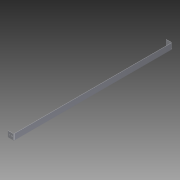
# Autodesk Inventor part: Climber Connector Bar
Saved by Autodesk Inventor 2014 SP1 (Build 180222100, 222)
## iProperties
Created: 2013-12-13
Part Number: Climber Connector Bar
Material: Aluminum 6061
Document SubType Name: Sheet Metal
Designer: Moses
Density: 2.71 g/cm^3
Appearance: Aluminum - Flat
Sheet Metal Rule: Default
Mass: 42.8559 g
Surface Area: 408.203 cm^2
Volume: 15.814 cm^3
Author: Moses
Autodesk Inventor part; units mm, degrees
ref_plane "YZ Plane" through (0, 0, 0) normal (1, 0, 0) x (0, 1, 0)
ref_plane "XZ Plane" through (0, 0, 0) normal (0, 1, 0) x (-1, 0, 0)
ref_plane "XY Plane" through (0, 0, 0) normal (0, 0, 1) x (1, 0, 0)
sketch "Sketch1" plane through (0, 0, 0) normal (0, 0, 1) x (1, 0, 0)
  line L0 (0, 0) -> (19.05, 0)
  line L1 (19.05, 0) -> (19.05, 19.05)
  line L2 (19.05, 19.05) -> (18.2563, 19.05)
  line L3 (18.2563, 19.05) -> (18.2563, 0.7938)
  line L4 (18.2563, 0.7938) -> (0, 0.7937)
  line L5 (0, 0.7937) -> (0, 0)
  dimension "d0" = 19.05
  dimension "d1" = 19.05
  dimension "d2" = 0.7937
  constraints: 12 end point, 3 horizontal, 3 vertical, 1 perpendicular
  measures "d0" distance of L0.start L0.end
  measures "d1" distance of L0.end L1.end
  measures "d2" distance of L1.end L2.end
extrude "Extrusion1" add sketch "Sketch1" along normal blind 260.35
sketch "Sketch2" plane through (0, 0, 260.35) normal (0, 0, 1) x (1, 0, 0)
  line L0 (0, 0) -> (19.05, 0) projected
  line L1 (19.05, 0) -> (19.05, 19.05) projected
  line L2 (19.05, 19.05) -> (18.2563, 19.05) projected
  line L3 (18.2563, 19.05) -> (18.2563, 0.7938) projected
  line L4 (18.2563, 0.7938) -> (18.2563, 0)
  constraints: 2 end point, 1 point on line, 1 vertical
extrude "Extrusion2" cut sketch "Sketch2" against normal blind 3.175
sketch "Sketch3" plane through (18.2563, 0, 259.5563) normal (0, 0, 1) x (1, 0, 0)
  line L0 (-18.2563, 0) -> (0, 0)
  line L1 (0, 0) -> (0, 19.05)
  line L2 (0, 19.05) -> (-18.2563, 19.05)
  line L3 (-18.2563, 19.05) -> (-18.2563, 0)
  constraints: 6 end point, 1 horizontal, 1 perpendicular, 1 vertical
edge flange "Flange1" height 19.05 angle 90 thickness 0.7937 bend radius 0.635 thickness toward (0, 0, 1) relief straight relief width 0.7937 relief depth 0.3969 edges at (9.1281, 0.7938, 260.35) wall of the first edge with corners at (0, 0, 259.5563) (18.2563, 0, 259.5563) (18.2562, 19.05, 259.5563) (0, 19.05, 259.5563)
bend "Bend1"
corner "Corner1"
sketch "Sketch4" plane through (0, 19.05, 260.35) normal (0, 0, 1) x (1, 0, 0)
  line L0 (0, -17.6213) -> (18.2563, -17.6213) projected
  line L1 (0, 0) -> (18.2563, 0) projected
  circle A0 centre (5.1594, -8.8106) radius 1.5875
  circle A1 centre (13.0969, -8.8106) radius 1.5875
  line L2 (5.1594, -8.8106) -> (13.0969, -8.8106) construction
  line L3 (9.1281, 0) -> (9.1281, -17.6213) construction
  point P0 (0, -19.05)
  point P1 (9.1281, -8.8106)
  dimension "d21" = 3.175
  dimension "d22" = 7.9375
  constraints: 4 end point, 4 midpoint, 2 centre point, 1 equal radius, 1 horizontal
  measures "d21" diameter of A0
  measures "d22" distance of L2.end L2.start
extrude "Extrusion3" cut sketch "Sketch4" against normal through all
mirror "Mirror1" about plane through (13.8989, 5.1511, 0) normal (0, 0, -1)
equation "\"d7\" = BendReliefWidth"
equation "\"d8\" = BendReliefDepth"
equation "\"d9\" = MinimumRemnant"
equation "\"d10\" = BendRadius"
equation "\"d14\" = CornerReliefSize"
equation "\"d15\" = GapSize"
equation "\"d16\" = JacobiRadiusSize"
equation "\"BendRadius\" = Thickness"
equation "\"BendReliefWidth\" = Thickness"
equation "\"BendReliefDepth\" = 0.5 * Thickness"
equation "\"CornerReliefSize\" = 4 * Thickness"
equation "\"MinimumRemnant\" = 2 * Thickness"
equation "\"TransitionRadius\" = BendRadius"
equation "\"JacobiRadiusSize\" = Thickness"
equation "\"GapSize\" = Thickness"
equation "\"Thickness\" = 0.79375"
body "Solid1"
